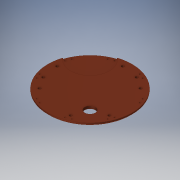
# Autodesk Inventor part: 4K sheild top
Saved by Autodesk Inventor 2018 (Build 220112000, 112)
## iProperties
Created: 2019-03-11
Part Number: 4K sheild top
Material: Copper
Document SubType Name: Modeling
Designer: Admin
Density: 8.94 g/cm^3
Appearance: Copper - Satin
Author: Admin
Autodesk Inventor part; units mm, degrees
ref_plane "YZ Plane" through (0, 0, 0) normal (1, 0, 0) x (0, 1, 0)
ref_plane "XZ Plane" through (0, 0, 0) normal (0, 1, 0) x (-1, 0, 0)
ref_plane "XY Plane" through (0, 0, 0) normal (0, 0, 1) x (1, 0, 0)
sketch "Sketch1" plane through (0, 0, 0) normal (0, 1, 0) x (-1, 0, 0)
  circle A0 centre (0, 0) radius 101.6
  dimension "d0" = 203.2
  constraints: 1 centre point, 1 coincident
  measures "d0" diameter of A0
extrude "Extrusion1" add sketch "Sketch1" along normal blind 6.35
sketch "Sketch3" plane through (0, 6.35, 0) normal (0, 1, 0) x (1, 0, 0)
  line L0 (0, 0) -> (87.9995, 36.4506) construction
  line L1 (0, 0) -> (95.25, 0) construction
  line L2 (87.9995, 36.4506) -> (90.4296, 30.584) construction
  point P0 (85.5695, 42.3172)
  point P1 (85.5695, 42.3172)
  dimension "d14" = 95.25
  dimension "d15" = 22.5
  dimension "d16" = 6.35
  dimension "d17" = 90
  constraints: 6 end point, 2 coincident, 1 equal length, 1 horizontal, 1 symmetric about line
  measures "d14" distance of L0.start L0.end
  measures "d15" angle of L1 L0
  measures "d16" distance of L0.end L2.end
  measures "d17" angle of L2 L0
hole "Hole2" at (90.4296, 6.35, -30.584) at (85.5695, 6.35, -42.3172) direction (0, -1, 0) diameter 3.81 depth 8.8646 tip angle 118 clearance for "Flat Head Machine Screw (82)" size "#6" standard "Ansi Unified Screw Threads"
pattern_circular "Circular Pattern2" count 8 over 360 about axis through (0, 0, 0) along (0, 1, 0) of "Hole2"
sketch "Sketch5" plane through (0, 0, 0) normal (0, -1, 0) x (1, 0, 0)
  circle A0 centre (0, 0) radius 101.6
  circle A1 centre (0, 0) radius 101.6
  circle A2 centre (0, 0) radius 98.425
  dimension "d31" = 196.85
  constraints: 3 centre point, 2 coincident, 2 concentric
  measures "d31" diameter of A2
extrude "Extrusion3" cut sketch "Sketch5" against normal blind 3.175
sketch "Sketch6" plane through (0, 6.35, 0) normal (0, 1, 0) x (1, 0, 0)
  line L0 (0, 0) -> (71.842, -71.842) construction
  line L1 (0, 0) -> (101.6, 0) construction
  line L2 (71.842, -71.842) -> (44.9013, -44.9013) construction
  circle A0 centre (44.9013, -44.9013) radius 12.7
  dimension "d39" = 101.6
  dimension "d40" = 45
  dimension "d41" = 38.1
  dimension "d42" = 25.4
  constraints: 6 end point, 1 centre point, 1 coincident, 1 equal length, 1 horizontal, 1 point on line
  measures "d39" distance of L0.start L0.end
  measures "d40" angle of L0 L1
  measures "d41" distance of L0.end L2.end
  measures "d42" diameter of A0
extrude "Extrusion4" cut sketch "Sketch6" against normal blind 25.4
sketch "Sketch8" plane through (0, 6.35, 0) normal (0, 1, 0) x (1, 0, 0)
  circle A0 centre (44.9013, -44.9013) radius 12.7 construction
  line L0 (44.9013, -44.9013) -> (-60.1677, 60.1677) construction
  line L1 (44.9013, -44.9013) -> (193.4913, -44.9013) construction
  circle A1 centre (-60.1677, 60.1677) radius 46.99
  point P0 (0, 0)
  dimension "d64" = 148.59
  dimension "d65" = 135
  dimension "d66" = 93.98
  constraints: 4 end point, 1 centre point, 1 coincident, 1 equal length, 1 horizontal
  measures "d64" distance of L0.start L0.end
  measures "d65" angle of L1 L0
  measures "d66" diameter of A1
sketch "Sketch7" plane through (0, 6.35, 0) normal (0, 1, 0) x (1, 0, 0)
  circle A0 centre (44.9013, -44.9013) radius 12.7 construction
  line L0 (44.9013, -44.9013) -> (0, 0) construction
  line L1 (44.9013, -44.9013) -> (-23.5283, 23.5283) construction
  line L2 (44.9013, -44.9013) -> (141.6753, -44.9013) construction
  circle A1 centre (-23.5283, 23.5283) radius 139.7 construction
  line L3 (-23.5283, 23.5283) -> (4.7102, 160.3445)
  line L4 (-23.5283, 23.5283) -> (116.1717, 23.5283) construction
  line L5 (-23.5283, 23.5283) -> (-160.3445, -4.7102)
  circle A2 centre (0, 0) radius 83.82 construction
  line L6 (0, 0) -> (-83.82, 0) construction
  line L7 (0, 0) -> (0, 83.82) construction
  line L8 (0, 0) -> (83.82, 0) construction
  line L9 (0, 0) -> (0, -83.82) construction
  dimension "d45" = 63.5
  dimension "d46" = 96.774
  dimension "d47" = 135
  dimension "d48" = 279.4
  dimension "d49" = 139.7
  dimension "d50" = 281.662
  dimension "d56" = 167.64
  constraints: 20 end point, 6 coincident, 4 horizontal, 4 point on circle, 2 centre point, 2 equal length, 2 perpendicular, 1 symmetric about line
  measures "d45" distance of L0.start L0.end
  measures "d46" distance of L0.start L1.end
  measures "d47" angle of L2 L1
  measures "d48" diameter of A1
  measures "d49" distance of L3.start L3.end
  measures "d56" diameter of A2
hole "Hole3" [suppressed]
extrude "Extrusion6" cut sketch "Sketch8" against normal blind 2.54
sketch "Sketch9" plane through (0, 6.35, 0) normal (0, 1, 0) x (1, 0, 0)
  circle A0 centre (0, 0) radius 86.36 construction
  line L0 (0, 0) -> (79.7862, -33.0485) construction
  line L1 (0, 0) -> (86.36, 0) construction
  line L2 (0, 0) -> (86.36, 0) construction
  line L3 (0, 0) -> (-6.9773, 86.0777) construction
  line L4 (0, 0) -> (86.36, 0) construction
  line L5 (0, 0) -> (-61.0657, 61.0657) construction
  line L6 (0, 0) -> (86.36, 0) construction
  line L7 (0, 0) -> (33.0485, 79.7862) construction
  line L8 (0, 0) -> (86.36, 0) construction
  line L9 (0, 0) -> (60.8117, 61.3187) construction
  line L10 (0, 0) -> (86.36, 0) construction
  circle A1 centre (30.584, 90.4296) radius 1.905 projected
  line L11 (0, 0) -> (30.584, 90.4296) construction
  circle A2 centre (42.3172, 85.5695) radius 1.905 projected
  line L12 (42.3172, 85.5695) -> (0, 0) construction
  point P0 (33.0485, -79.7862)
  point P1 (-86.0777, 6.9773)
  point P2 (-79.7862, -33.0485)
  point P3 (-79.7862, -33.0485)
  point P4 (-86.0777, 6.9773)
  point P5 (-61.3187, -60.8117)
  dimension "d71" = 172.72
  dimension "d72" = 22.5
  dimension "d76" = 135
  dimension "d86" = 45.238
  dimension "d88" = 94.634
  dimension "d101" = 67.5
  constraints: 26 end point, 6 coincident, 6 horizontal, 6 symmetric about line, 5 point on circle, 4 equal length, 1 centre point, 1 other
  measures "d71" diameter of A0
  measures "d72" angle of L0 L1
  measures "d76" angle of L6 L5
  measures "d86" angle of L10 L9
  measures "d88" angle of L1 L3
  measures "d101" angle of L1 L7
hole "Hole4" at (79.7862, 6.35, 33.0485) at (-6.9773, 6.35, -86.0777) at (33.0485, 6.35, -79.7862) at (33.0485, 6.35, 79.7862) at (-79.7862, 6.35, 33.0485) at (-86.0777, 6.35, -6.9773) at (60.8117, 6.35, -61.3187) at (-61.3187, 6.35, 60.8117) direction (0, -1, 0) diameter 6.7564 depth 25.4 tip angle 118 clearance for "Flat Head Machine Screw (82)" size "1/4" standard "Ansi Unified Screw Threads"
body "Solid1"
